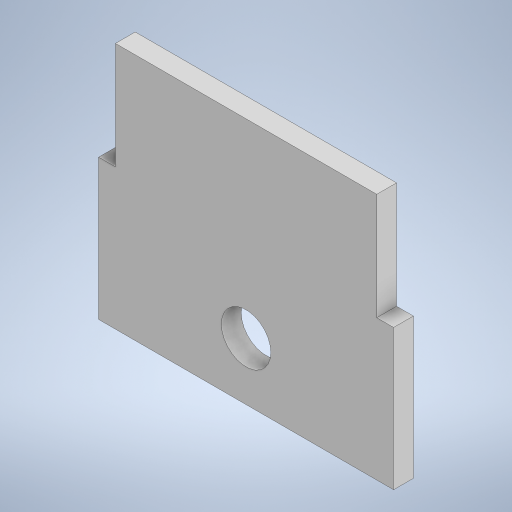
# Autodesk Inventor part: frontPlate
Saved by Autodesk Inventor 2023 (Build 270158030, 158C)
## iProperties
Created: 2022-06-04
Part Number: frontPlate
Material: Generic
Document SubType Name: Modeling
Designer: snobo
Density: 1 g/cm^3
Appearance: Default
Author: snobo
Autodesk Inventor part; units mm, degrees
ref_plane "YZ Plane" through (0, 0, 0) normal (1, 0, 0) x (0, 1, 0)
ref_plane "XZ Plane" through (0, 0, 0) normal (0, 1, 0) x (-1, 0, 0)
ref_plane "XY Plane" through (0, 0, 0) normal (0, 0, 1) x (1, 0, 0)
sketch "Sketch1" plane through (0, 0, 0) normal (0, 0, 1) x (1, 0, 0)
  line L0 (-74.5, -62.5) -> (74.5, -62.5)
  line L1 (74.5, -62.5) -> (74.5, 8.5)
  line L2 (66, 62.5) -> (-66, 62.5)
  line L3 (-74.5, 8.5) -> (-74.5, -62.5)
  line L4 (-74.5, -62.5) -> (74.5, 62.5) construction
  line L5 (74.5, -62.5) -> (-74.5, 62.5) construction
  line L6 (-74.5, 8.5) -> (-66, 8.5)
  line L7 (-66, 8.5) -> (-66, 62.5)
  line L8 (74.5, 8.5) -> (66, 8.5)
  line L9 (66, 8.5) -> (66, 62.5)
  point P0 (0, 0)
  dimension "d0" = 149
  dimension "d1" = 125
  dimension "d5" = 54
  dimension "d6" = 8.5
  constraints: 20 end point, 3 horizontal, 3 perpendicular, 2 equal length, 2 midpoint, 2 parallel
  measures "d0" distance of L0.start L0.end
  measures "d1" distance of L4.end L0.end
  measures "d5" distance of L6.end L2.end
  measures "d6" distance of L3.start L6.end
extrude "Extrusion1" add sketch "Sketch1" against normal blind 10
sketch "Sketch2" plane through (0, 0, -10) normal (0, 0, -1) x (-1, 0, 0)
  circle A0 centre (0, -33.5) radius 27.5
  circle A1 centre (0, -33.5) radius 23
  line L0 (-74.5, -62.5) -> (74.5, -62.5) projected
  point P0 (0, 0)
  dimension "d9" = 55
  dimension "d10" = 46
  dimension "d11" = 29
  constraints: 2 centre point, 1 coincident
  measures "d9" diameter of A0
  measures "d10" diameter of A1
  measures "d11" distance from line of A0.centre L0
extrude "Extrusion2" cut sketch "Sketch2" against normal blind 5
sketch "Sketch3" plane through (0, -33.5, -10) normal (0, 0, -1) x (-1, 0, 0)
  circle A0 centre (0, 0) radius 12.5
  point P0 (0, 33.5)
  dimension "d14" = 25
  constraints: 1 centre point
  measures "d14" diameter of A0
extrude "Extrusion3" cut sketch "Sketch3" against normal through all
body "Solid1"
